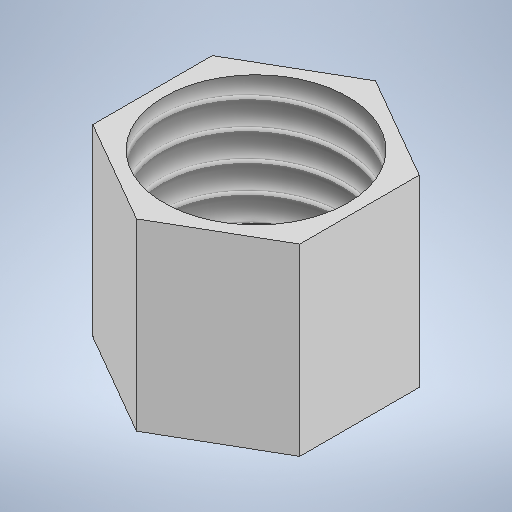
# Autodesk Inventor part: 124
Saved by Autodesk Inventor 2025.1 (Build 291241000, 241)
## iProperties
Created: 2024-08-21
Part Number: 124
Material: Generisch
Document SubType Name: Modeling
Designer: ffogue
Density: 1 g/cm^3
Appearance: Vorgabe
Author: ffogue
Autodesk Inventor part; units mm, degrees
ref_plane "YZ Plane" through (0, 0, 0) normal (1, 0, 0) x (0, 1, 0)
ref_plane "XZ Plane" through (0, 0, 0) normal (0, 1, 0) x (-1, 0, 0)
ref_plane "XY Plane" through (0, 0, 0) normal (0, 0, 1) x (1, 0, 0)
sketch "Sketch1" plane through (0, 0, 0) normal (0, 0, 1) x (1, 0, 0)
  line L0 (0, 6.5) -> (5.6292, 3.25)
  line L1 (5.6292, 3.25) -> (5.6292, -3.25)
  line L2 (5.6292, -3.25) -> (0, -6.5)
  line L3 (0, -6.5) -> (-5.6292, -3.25)
  line L4 (-5.6292, -3.25) -> (-5.6292, 3.25)
  line L5 (-5.6292, 3.25) -> (0, 6.5)
  point P0 (0, 0)
  point P1 (0, 0)
  dimension "d0" = 13
  constraints: 12 end point, 1 coincident, 13 other
  measures "d0" distance of L2.end L0.start
extrude "Extrusion1" add sketch "Sketch1" against normal blind 10
sketch "Sketch2" plane through (0, 0, 0) normal (0, 0, 1) x (1, 0, 0)
  point P0 (0, 0)
  point P1 (0, 0)
  constraints: 1 coincident
hole "Hole1" at (0, 0, 0) direction (0, 0, -1) diameter 10 depth 7
thread "Thread1" size "M10x1.5" class "6H" standard "ISO Metric profile" length 10
sketch "Sketch3" plane through (0, 0, -10) normal (0, 0, -1) x (-1, 0, 0)
  point P0 (0, 0)
  point P1 (0, 0)
  constraints: 1 coincident
hole "Hole2" at (0, 0, -10) direction (0, 0, 1) diameter 6 depth 4
body "Solid1"
